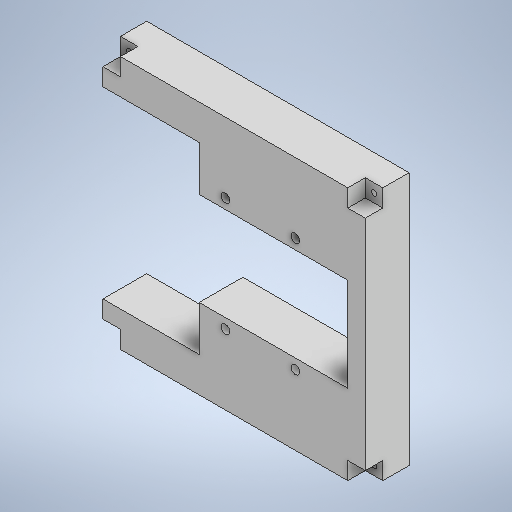
# Autodesk Inventor part: RobotBase
Saved by Autodesk Inventor 2025.3 (Build 293356000, 356)
## iProperties
Created: 2025-04-27
Part Number: RobotBase
Material: 일반
Document SubType Name: Modeling
Designer: SEON
Density: 1 g/cm^3
Appearance: 기본값
Author: SEON
## iProperties of the stored document RobotBase_3D 인쇄.ipt
Created: 2025-05-08
Part Number: RobotBase_3D 인쇄
Material: 일반
Document SubType Name: Modeling
Designer: SEON
Density: 1 g/cm^3
Appearance: 기본값
Author: SEON
Autodesk Inventor part; units mm, degrees
ref_plane "YZ Plane" through (0, 0, 0) normal (1, 0, 0) x (0, 1, 0)
ref_plane "XZ Plane" through (0, 0, 0) normal (0, 1, 0) x (-1, 0, 0)
ref_plane "XY Plane" through (0, 0, 0) normal (0, 0, 1) x (1, 0, 0)
sketch "스케치1" plane through (0, 0, 0) normal (0, 0, 1) x (1, 0, 0)
  line L0 (0, 0) -> (300, 0)
  line L1 (300, 0) -> (300, 290)
  line L2 (300, 290) -> (0, 290)
  line L3 (0, 290) -> (0, 0)
  line L4 (300, 270) -> (245, 270)
  line L5 (245, 270) -> (245, 165)
  line L6 (245, 165) -> (300, 165)
  line L7 (300, 165) -> (300, 270)
  line L8 (150, 290) -> (150, 145)
  line L9 (0, 270) -> (55, 270)
  line L10 (55, 270) -> (55, 165)
  line L11 (55, 165) -> (0, 165)
  line L12 (300, 145) -> (150, 145)
  line L13 (300, 20) -> (245, 20)
  line L14 (245, 20) -> (245, 125)
  line L15 (245, 125) -> (300, 125)
  line L16 (55, 125) -> (0, 125)
  line L17 (55, 20) -> (55, 125)
  line L18 (0, 20) -> (55, 20)
  line L19 (0, 145) -> (150, 145)
  circle A0 centre (5, 150) radius 1.5
  circle A1 centre (145, 150) radius 1.5
  circle A2 centre (5, 285) radius 1.5
  circle A3 centre (145, 285) radius 1.5
  point P0 (300, 165)
  point P1 (0, 165)
  dimension "d0" = 290
  dimension "d1" = 300
  dimension "d12" = 105
  dimension "d13" = 55
  dimension "d14" = 20
  dimension "d18" = 5
  dimension "d19" = 3
  dimension "d20" = 5
  dimension "d21" = 5
  dimension "d22" = 5
  constraints: 40 end point, 12 symmetric about line, 4 centre point, 4 horizontal, 4 parallel, 3 equal radius, 3 midpoint, 2 horizontal alignment, 2 perpendicular, 2 vertical alignment, 1 point on line, 1 vertical
  measures "d0" distance of L2.end L0.start
  measures "d1" distance of L0.start L0.end
  measures "d12" distance of L4.end L5.end
  measures "d13" distance of L5.end L6.end
  measures "d14" distance between parallel lines of L2 L4
  measures "d18" distance from line of L19 A0.centre
  measures "d19" diameter of A0
  measures "d20" distance from line of L3 A0.centre
  measures "d21" horizontal distance of L8.end A1.centre
  measures "d22" distance from line of L2 A3.centre
extrude "돌출1" add sketch "스케치1" along normal blind 25 contours L3 L11 L10 L9 L2 L8 L19
sketch "스케치3" plane through (0, 0, 25) normal (0, 0, 1) x (1, 0, 0)
  line L0 (55, 165) -> (0, 165) projected
  line L1 (0, 165) -> (0, 145) projected
  line L2 (0, 145) -> (150, 145) projected
  line L3 (150, 145) -> (150, 290) projected
  line L4 (150, 290) -> (0, 290) projected
  line L5 (0, 290) -> (0, 270) projected
  line L6 (0, 270) -> (55, 270) projected
  line L7 (55, 270) -> (55, 165) projected
  circle A0 centre (145, 285) radius 1.5 projected
  circle A1 centre (5, 285) radius 1.5 projected
  circle A2 centre (145, 150) radius 1.5 projected
  circle A3 centre (5, 150) radius 1.5 projected
  line L8 (140, 145) -> (140, 290)
  line L9 (140, 155) -> (150, 155)
  line L10 (140, 280) -> (150, 280)
  line L11 (0, 155) -> (10, 155)
  line L12 (10, 155) -> (10, 145)
  line L13 (0, 280) -> (10, 280)
  line L14 (10, 280) -> (10, 290)
  point P0 (0, 0)
  dimension "d23" = 10
  dimension "d24" = 10
  dimension "d25" = 10
  constraints: 14 end point, 8 point on line, 7 perpendicular, 2 horizontal, 2 midpoint
  measures "d23" distance between parallel lines of L4 L10
  measures "d24" distance between parallel lines of L2 L9
  measures "d25" distance between parallel lines of L3 L8
extrude "돌출3" cut sketch "스케치3" against normal blind 10 contours L11 L12 L2 L1 | L5 L4 L14 L13 | L8 L9 L3 L2 | L4 L3 L10 L8
sketch "스케치4" plane through (55, 165, 0) normal (-1, 0, 0) x (0, 0, 1)
  line L0 (22, 11) -> (22, 94)
  line L1 (22, 94) -> (0, 94)
  line L2 (0, 105) -> (0, 0) projected
  line L3 (0, 0) -> (25, 0) projected
  line L4 (25, 105) -> (25, 0) projected
  line L5 (0, 105) -> (25, 105) projected
  line L6 (22, 11) -> (0, 11)
  circle A0 centre (14.25, 17) radius 2.5
  circle A1 centre (14.25, 88) radius 2.5
  line L7 (0, 25.75) -> (0, 79.25)
  line L8 (0, 25.75) -> (25, 25.75)
  line L9 (0, 79.25) -> (25, 79.25)
  line L10 (6.5, 11) -> (6.5, 94)
  point P0 (0, -165)
  point P1 (22, 52.5)
  point P2 (25, 52.5)
  point P3 (0, 52.5)
  point P4 (6.5, 79.25)
  point P5 (22, 79.25)
  point P6 (6.5, 25.75)
  point P7 (22, 25.75)
  dimension "d28" = 83
  dimension "d30" = 5
  dimension "d31" = 5
  dimension "d33" = 6
  dimension "d34" = 6
  dimension "d35" = 53.5
  dimension "d36" = 15.5
  dimension "d37" = 7.75
  dimension "d39" = 3
  constraints: 14 end point, 6 point on line, 5 perpendicular, 4 midpoint, 2 centre point, 2 horizontal alignment, 2 vertical, 1 vertical alignment
  measures "d28" distance of L0.start L0.end
  measures "d30" diameter of A0
  measures "d31" diameter of A1
  measures "d33" distance from line of L6 A0.centre
  measures "d34" distance from line of L1 A1.centre
  measures "d35" distance of L7.start L7.end
  measures "d36" distance between parallel lines of L0 L10
  measures "d37" distance from line of L0 A0.centre
  measures "d39" distance between parallel lines of L4 L0
extrude "돌출5" cut sketch "스케치4" against normal blind 85 contours L8 L10 L9 L0 | L0 L9 L4 L8 | L8 L2 L9 L10
sketch "스케치5" plane through (0, 0, 25) normal (0, 0, 1) x (1, 0, 0)
  line L0 (55, 244.25) -> (140, 244.25) projected
  line L1 (140, 244.25) -> (140, 190.75) projected
  line L2 (140, 190.75) -> (55, 190.75) projected
  line L3 (55, 190.75) -> (55, 165) projected
  line L4 (55, 165) -> (0, 165) projected
  line L5 (0, 165) -> (0, 155) projected
  line L6 (0, 155) -> (10, 155) projected
  line L7 (10, 155) -> (10, 145) projected
  line L8 (10, 145) -> (140, 145) projected
  line L9 (140, 145) -> (140, 155) projected
  line L10 (140, 155) -> (150, 155) projected
  line L11 (150, 155) -> (150, 280) projected
  line L12 (150, 280) -> (140, 280) projected
  line L13 (140, 280) -> (140, 290) projected
  line L14 (140, 290) -> (10, 290) projected
  line L15 (10, 290) -> (10, 280) projected
  line L16 (10, 280) -> (0, 280) projected
  line L17 (0, 280) -> (0, 270) projected
  line L18 (0, 270) -> (55, 270) projected
  line L19 (55, 270) -> (55, 244.25) projected
  circle A0 centre (70, 185) radius 2.5
  circle A1 centre (70, 250) radius 2.5
  circle A2 centre (110, 185) radius 2.5
  circle A3 centre (110, 250) radius 2.5
  point P0 (0, 0)
  point P1 (140, 217.5)
  dimension "d47" = 15
  dimension "d48" = 65
  dimension "d49" = 32.5
  dimension "d50" = 5
  dimension "d51" = 65
  dimension "d52" = 5
  dimension "d53" = 40
  constraints: 4 centre point, 2 equal radius, 2 vertical alignment, 1 horizontal alignment, 1 midpoint
  measures "d47" distance from line of L3 A0.centre
  measures "d48" distance of A1.centre A0.centre
  measures "d49" vertical distance of point (140, 217.5) A0.centre
  measures "d50" diameter of A0
  measures "d51" distance of A3.centre A2.centre
  measures "d52" diameter of A2
  measures "d53" distance of A0.centre A2.centre
extrude "돌출7" cut sketch "스케치5" against normal through all contours A0 | A1 | A2 | A3
equation "\"d20\" = d18"
equation "\"d21\" = d20"
equation "\"d22\" = d21"
equation "\"d37\" = 0.5 * d36"
equation "\"d49\" = 0.5 * d48"
